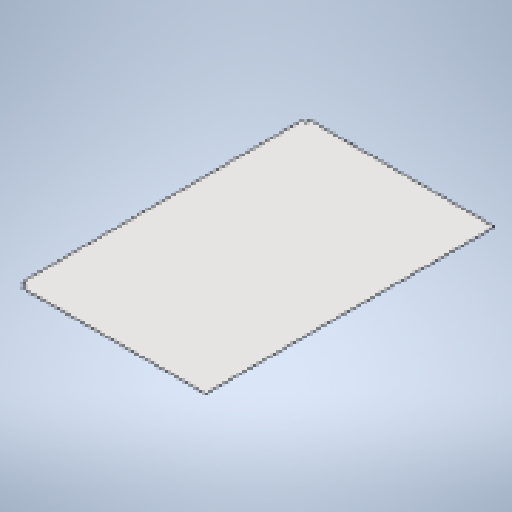
# Autodesk Inventor part: SLM-frame 1.1 floor sheet 4_CPY
Saved by Autodesk Inventor 2025.3 (Build 293356030, 356C)
## iProperties
Created: 2025-10-28
Part Number: SLM-frame 1.1 floor sheet 4_CPY
Material: Stainless Steel
Document SubType Name: Sheet Metal
Designer: admin
Stock Number: 1.4
Mass: 280.619 g
Surface Area: 364.406 cm^2
Volume: 35.0774 cm^3
Density: 8 g/cm^3
Flat Pattern Width: 150 cm
Flat Pattern Length: 230 cm
Flat Pattern Area: 34500 cm^2
Sheet Metal Rule: AISI304 3mm Die 32
Sheet Metal Width: 1500,000 mm
Sheet Metal Length: 2300,000 mm
Sheet Metal Area: 3450000,000 mm^2
Appearance: Default
Author: admin
Autodesk Inventor part; units mm, degrees
ref_plane "YZ Plane" through (0, 0, 0) normal (1, 0, 0) x (0, 1, 0)
ref_plane "XZ Plane" through (0, 0, 0) normal (0, 1, 0) x (-1, 0, 0)
ref_plane "XY Plane" through (0, 0, 0) normal (0, 0, 1) x (1, 0, 0)
sketch "Sketch1" plane through (0, 0, 0) normal (0, 0, 1) x (1, 0, 0)
  line L0 (0, 0) -> (-1500, 0)
  line L1 (-1500, 0) -> (-1500, -2300)
  line L2 (-1500, -2300) -> (0, -2300)
  line L3 (0, -2300) -> (0, 0)
  line L4 (0, 0) -> (-35, 0)
  line L5 (-35, 0) -> (-35, -35)
  line L6 (-35, -35) -> (0, -35)
  line L7 (0, -35) -> (0, 0)
  line L8 (0, -2300) -> (-35, -2300)
  line L9 (-35, -2300) -> (-35, -2265)
  line L10 (-35, -2265) -> (0, -2265)
  line L11 (0, -2265) -> (0, -2300)
  line L12 (-1500, 0) -> (-1465, 0)
  line L13 (-1465, 0) -> (-1465, -35)
  line L14 (-1465, -35) -> (-1500, -35)
  line L15 (-1500, -35) -> (-1500, 0)
  line L16 (-1500, -2300) -> (-1465, -2300)
  line L17 (-1465, -2300) -> (-1465, -2265)
  line L18 (-1465, -2265) -> (-1500, -2265)
  line L19 (-1500, -2265) -> (-1500, -2300)
  line L20 (-1435, -2300) -> (-1345, -2300)
  line L21 (-1345, -2300) -> (-1345, -2265)
  line L22 (-1345, -2265) -> (-1435, -2265)
  line L23 (-1435, -2265) -> (-1435, -2300)
  line L24 (-1435, 0) -> (-1345, 0)
  line L25 (-1345, 0) -> (-1345, -35)
  line L26 (-1345, -35) -> (-1435, -35)
  line L27 (-1435, -35) -> (-1435, 0)
  point P0 (0, -35)
  point P1 (0, -2265)
  point P2 (-1345, 0)
  dimension "d22" = 1500
  dimension "d23" = 2300
  dimension "d24" = 35
  dimension "d25" = 35
  dimension "d28" = 90
  dimension "d29" = 1310
  measures "d22" distance of L2.end L1.end
  measures "d23" distance of L1.end L0.end
  measures "d24" distance of L6.end L5.end
  measures "d25" distance of L5.end L4.end
  measures "d28" distance of L25.end L26.end
  measures "d29" distance between parallel lines of L5 L25
extrude "Plate1" add sketch "Sketch1" along normal blind 3 contours L3 L6 L5 L0 | L5 L6 L3 L10 L9 L2 L21 L22 L23 L17 L18 L1 L14 L13 L0 L27 L26 L25 | L25 L26 L27 L0 | L3 L2 L9 L10 | L2 L23 L22 L21
sketch "Sketch5" plane through (0, 0, 3) normal (0, 0, 1) x (1, 0, 0)
  line L0 (-1195, 0) -> (-1190, 0)
  line L1 (-1185, 0) -> (-1180, 0)
  circle A0 centre (-1200, 0) radius 2.5
  line L2 (-1170, 0) -> (-1170, -5)
  line L3 (-1165, 0) -> (-1163.6916, -4.1277)
  arc A1 (-1163.6916, -4.1277) -> (-1161.3084, -4.1277) centre (-1162.5, -3.75) ccw
  line L4 (-1165, 0) -> (-1160, 0)
  line L5 (-1170, 0) -> (-1165, 0) construction
  line L6 (-1160, 0) -> (-1155, 0) construction
  line L7 (-1161.3084, -4.1277) -> (-1160, 0)
  line L8 (-1155, -5) -> (-1155, 0)
  line L9 (-1155, 0) -> (-1150, 0)
  line L10 (-1150, 0) -> (-1150, -5)
  line L11 (-1150, -5) -> (-1155, -5)
  line L12 (-1150, -2.5) -> (-1145, -2.5) construction
  line L13 (-1180, -5) -> (-1185, -5)
  line L14 (-1170, -5) -> (-1175, -5)
  line L15 (-1180, -2.5) -> (-1175, -2.5) construction
  line L16 (-1190, -2.5) -> (-1185, -2.5) construction
  line L17 (-1175, 0) -> (-1170, 0)
  line L18 (-1175, -5) -> (-1175, 0)
  line L19 (-1180, 0) -> (-1180, -5)
  line L20 (-1185, -5) -> (-1185, 0)
  line L21 (-1190, 0) -> (-1190, -5)
  line L22 (-1195, -5) -> (-1195, 0)
  line L23 (-1190, -5) -> (-1195, -5)
  line L24 (-1145, -5) -> (-1145, 0)
  line L25 (-1140, -5) -> (-1145, -5)
  line L26 (-1145, 0) -> (-1140, 0)
  line L27 (-1140, 0) -> (-1140, -5)
  line L28 (-1140, -2.5) -> (-1135, -2.5) construction
  line L29 (-1135, -5) -> (-1135, 0)
  line L30 (-1135, 0) -> (-1130, 0)
  line L31 (-1130, 0) -> (-1130, -5)
  line L32 (-1130, -5) -> (-1135, -5)
  line L33 (-1465, 0) -> (0, 0) projected
  line L34 (-1120, -5) -> (-1125, -5)
  line L35 (-1125, -5) -> (-1125, 0)
  line L36 (-1120, 0) -> (-1120, -5)
  line L37 (-1125, 0) -> (-1120, 0)
  line L38 (-1125, -2.5) -> (-1130, -2.5)
  point P0 (-1162.5, 0)
  point P1 (-1500, 0)
  point P2 (-1122.5, 0)
  point P3 (-1120, 0)
  point P4 (-1125, 0)
  dimension "d30" = 5
  dimension "d31" = 5
  dimension "d32" = 1.25
  dimension "d33" = 5
  dimension "d34" = 5
  dimension "d35" = 5
  dimension "d36" = 5
  dimension "d37" = 5
  dimension "d38" = 300
  constraints: 76 end point, 14 parallel, 13 horizontal, 12 equal length, 12 midpoint, 7 perpendicular, 5 collinear, 3 point on line, 3 tangent, 2 centre point, 2 point on circle, 1 vertical alignment
  measures "d30" distance of L21.end L23.end
  measures "d31" distance of L23.end L0.start
  measures "d32" radius of A1
  measures "d33" distance of L5.end L4.end
  measures "d34" distance of L10.end L8.start
  measures "d35" distance of L8.start L6.end
  measures "d36" diameter of A0
  measures "d37" distance of A0.centre L0.start
  measures "d38" distance of point (-1500, 0) A0.centre
extrude "Cut1" cut sketch "Sketch5" against normal blind 3 contours L33 A0 | A0 L33 | L8 L9 L10 L11 | L24 L26 L27 L25 | L29 L30 L31 L32 | L33 L36 L34 L35
equation "\"d24\" = d25"
equation "\"d32\" = 0.25 * d30"
equation "\"d39\" = Thickness"
equation "\"d2\" = Thickness"
equation "\"BendReliefWidth\" = Thickness"
equation "\"BendReliefDepth\" = 0.5 * Thickness"
equation "\"CornerReliefSize\" = 4 * Thickness"
equation "\"MinimumRemnant\" = 2 * Thickness"
equation "\"TransitionRadius\" = BendRadius"
equation "\"JacobiRadiusSize\" = BendRadius"
equation "\"GapSize\" = Thickness"
equation "\"Thickness\" = 3"
equation "\"BendRadius\" = 5"
body "Solid1"
